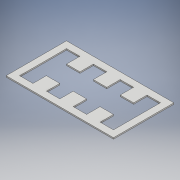
# Autodesk Inventor part: P2-4
Saved by Autodesk Inventor 2017 (Build 210142000, 142)
## iProperties
Created: 2017-02-09
Part Number: P2-4
Material: Generic
Document SubType Name: Modeling
Designer: Schaffel
Density: 1 g/cm^3
Appearance: Default
Author: Schaffel
Autodesk Inventor part; units mm, degrees
ref_plane "YZ Plane" through (0, 0, 0) normal (1, 0, 0) x (0, 1, 0)
ref_plane "XZ Plane" through (0, 0, 0) normal (0, 1, 0) x (-1, 0, 0)
ref_plane "XY Plane" through (0, 0, 0) normal (0, 0, 1) x (1, 0, 0)
sketch "Sketch1" plane through (0, 0, 0) normal (0, 0, 1) x (1, 0, 0)
  line L0 (0, 0) -> (160, 0)
  line L1 (160, 0) -> (160, 90)
  line L2 (160, 90) -> (0, 90)
  line L3 (0, 90) -> (0, 0)
  line L4 (10, 10) -> (30, 10)
  line L5 (30, 10) -> (30, 30)
  line L6 (30, 30) -> (50, 30)
  line L7 (50, 30) -> (50, 10)
  line L8 (50, 10) -> (70, 10)
  line L9 (70, 10) -> (70, 30)
  line L10 (70, 30) -> (90, 30)
  line L11 (90, 30) -> (90, 10)
  line L12 (90, 10) -> (110, 10)
  line L13 (110, 10) -> (110, 30)
  line L14 (110, 30) -> (130, 30)
  line L15 (130, 30) -> (130, 10)
  line L16 (130, 10) -> (150, 10)
  line L17 (150, 10) -> (150, 80)
  line L18 (150, 80) -> (130, 80)
  line L19 (130, 80) -> (130, 60)
  line L20 (130, 60) -> (110, 60)
  line L21 (110, 60) -> (110, 80)
  line L22 (90, 80) -> (110, 80)
  line L23 (90, 80) -> (90, 60)
  line L24 (70, 60) -> (90, 60)
  line L25 (70, 60) -> (70, 80)
  line L26 (70, 80) -> (50, 80)
  line L27 (50, 80) -> (50, 60)
  line L28 (50, 60) -> (30, 60)
  line L29 (30, 60) -> (30, 80)
  line L30 (30, 80) -> (10, 80)
  line L31 (10, 80) -> (10, 10)
  constraints: 64 end point, 32 point on line, 16 perpendicular, 2 horizontal
extrude "Extrusion1" add sketch "Sketch1" along normal blind 2
body "Solid1"
